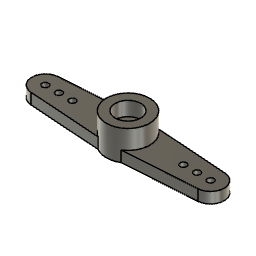
サーボホーン3 v2 (Autodesk Fusion 360 design; units mm, degrees)
Autodesk Fusion 360 part; units mm, degrees
note: some values were not read from the file. Set by a fixed rule: which sketch regions a step uses.
sketch "スケッチ1" plane through (0, 0, 0) normal (0, 0, 1) x (1, 0, 0)
  line L0 (2.1072, 3.4) -> (-2.1072, 3.4) construction
  line L1 (-2.1071, -3.4) -> (2.1071, -3.4) construction
  line L2 (17.7, 3.4) -> (-17.7, 3.4) construction
  line L3 (-17.7, 3.4) -> (-17.7, -3.4) construction
  line L4 (-17.7, -3.4) -> (17.7, -3.4) construction
  line L5 (17.7, -3.4) -> (17.7, 3.4) construction
  line L6 (17.7, 3.4) -> (-17.7, -3.4) construction
  line L7 (-17.7, 3.4) -> (17.7, -3.4) construction
  line L8 (-2.1072, 3.4) -> (-15.3703, 2.4942)
  line L9 (-2.1071, -3.4) -> (-15.3703, -2.4942)
  line L10 (2.1072, 3.4) -> (15.3703, 2.4942)
  line L11 (2.1071, -3.4) -> (15.3703, -2.4942)
  arc A0 (-15.3703, 2.4942) -> (-15.3703, -2.4942) centre (-15.2, 0) ccw
  arc A1 (15.3703, -2.4942) -> (15.3703, 2.4942) centre (15.2, 0) ccw
  arc A2 (2.1072, 3.4) -> (-2.1072, 3.4) centre (0, 0) ccw
  arc A3 (-2.1072, 3.4) -> (-2.1071, -3.4) centre (0, 0) ccw
  arc A4 (2.1071, -3.4) -> (2.1072, 3.4) centre (0, 0) ccw
  arc A5 (-2.1071, -3.4) -> (2.1071, -3.4) centre (0, 0) ccw
  line L12 (-2.1072, 3.4) -> (2.1072, 3.4)
  line L13 (-2.1071, -3.4) -> (2.1071, -3.4)
  circle A6 centre (-15.2, 0) radius 0.6
  circle A7 centre (-12.7, 0) radius 0.6
  circle A8 centre (-10.2, 0) radius 0.6
  line L14 (0, 1.75) -> (0, 22.5) construction
  circle A9 centre (10.2, 0) radius 0.6
  circle A10 centre (12.7, 0) radius 0.6
  circle A11 centre (15.2, 0) radius 0.6
  dimension "d1" = 8
  dimension "d5" = 6.8
  dimension "d6" = 35.4
  dimension "d7" = 6.8
  dimension "d8" = 2.5
  dimension "d9" = 2.5
  dimension "d10" = 1.2
  dimension "d11" = 2.5
  dimension "d14" = 2.5
  dimension "d15" = 0
  constraint coincident A2.centre A3.centre
  constraint horizontal L0
  constraint parallel L0 L1
  constraint coincident L1.end A3
  constraint horizontal L2
  constraint perpendicular L2 L3
  constraint parallel L2 L4
  constraint parallel L3 L5
  constraint coincident L6 A2.centre
  constraint coincident L7 A2.centre
  constraint tangent L9 A0
  constraint tangent L10 A1
  constraint tangent L5 A1
  constraint tangent L11 A1
  constraint tangent L3 A0
  constraint tangent L8 A0
  constraint midpoint L3 A0
  constraint midpoint L5 A1
  constraint concentric A2 A3
  constraint concentric A3 A4
  constraint concentric A3 A5
  constraint concentric A0 A6
  constraint symmetric A6 L14 A11
  constraint symmetric A7 L14 A10
  constraint symmetric A8 L14 A9
  measures "d1" diameter of A3
  measures "d5" distance of L0 L1
  measures "d6" distance of L3.end L4.end
  measures "d7" distance of L2.end L3.end
  measures "d8" radius of A0
  measures "d9" radius of A1
  measures "d10" diameter of A6
  measures "d11" distance of L3 A0.centre
extrude "押し出し1" add sketch "スケッチ1" along normal blind 5.5 contours A3 A4 L12 L13 | A2 L12 | A5 L13 makes body 1
extrude "押し出し2" add sketch "スケッチ1" along normal blind 2 contours L8 L9 A0 A3 | L10 L11 A1 A4 bodies 1
sketch "スケッチ2" plane through (0, 0, 5.5) normal (0, 0, 1) x (-1, 0, 0)
  circle A0 centre (0, 0) radius 4
  circle A1 centre (0, 0) radius 1
  circle A2 centre (0, 0) radius 2.35
  dimension "d23" = 2
  dimension "d24" = 4.7
  constraint coincident A0.centre A1.centre
  measures "d23" diameter of A1
  measures "d24" diameter of A2
extrude "押し出し3" cut sketch "スケッチ2" against normal through all contours A1 bodies 1
extrude "押し出し4" cut sketch "スケッチ2" against normal blind 2.6 contours A2 bodies 1
sketch "スケッチ3" plane through (0, 0, 0) normal (0, 0, 1) x (1, 0, 0)
  circle A0 centre (0, 0) radius 3.1
  dimension "d28" = 6.2
  constraint coincident A0.centre origin
  measures "d28" diameter of A0
extrude "押し出し5" cut sketch "スケッチ3" along normal blind 2.1 bodies 1
copy_body "ボディ -> コンポーネント1" bodies 1 removing the originals makes body 2 in component "Component'"
component "Component'" placed x (1, 0, 0) y (0, 1, 0) z (0, 0, 1) at (0, 0, 0)
